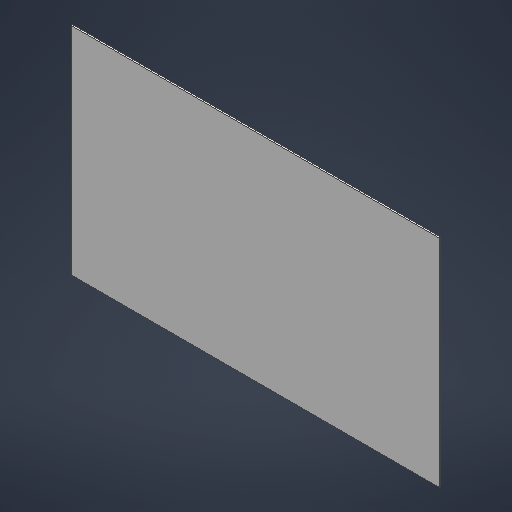
# Autodesk Inventor part: Floor
Saved by Autodesk Inventor 2026.2 (Build 302298000, 298)
## iProperties
Created: 2025-11-24
Part Number: Floor
Material: Genérico
Document SubType Name: Modeling
Designer: USUARIO
Density: 1 g/cm^3
Appearance: Valor por defecto
Author: USUARIO
Autodesk Inventor part; units mm, degrees
ref_plane "YZ Plane" through (0, 0, 0) normal (1, 0, 0) x (0, 1, 0)
ref_plane "XZ Plane" through (0, 0, 0) normal (0, 1, 0) x (-1, 0, 0)
ref_plane "XY Plane" through (0, 0, 0) normal (0, 0, 1) x (1, 0, 0)
sketch "Boceto1" plane through (0, 0, 0) normal (0, 0, 1) x (1, 0, 0)
  line L0 (-11500, 6750) -> (11500, 6750)
  line L1 (11500, 6750) -> (11500, -6750)
  line L2 (11500, -6750) -> (-11500, -6750)
  line L3 (-11500, -6750) -> (-11500, 6750)
  point P0 (0, 0)
  dimension "d0" = 23000
  dimension "d1" = 13500
  dimension "d2" = 11500
  dimension "d3" = 6750
  constraints: 8 end point, 2 parallel, 1 horizontal, 1 perpendicular
  measures "d0" distance of L0.start L0.end
  measures "d1" distance of L2.end L0.start
  measures "d2" distance from line of L3 point (0, 0)
  measures "d3" distance from line of L0 point (0, 0)
extrude "Extrusión1" add sketch "Boceto1" along normal blind 100
equation "\"d2\" = 0.5 * d0"
equation "\"d3\" = 0.5 * d1"
